Autodesk Fusion 360 part; units mm, degrees
note: some values were not read from the file. Chosen so that the rebuilt part matches the saved one: which bodies a step acts on; which face or edge a step refers to. Set by a fixed rule: which sketch regions a step uses.
(part 2 of 2)
sketch "Sketch34" plane through (0, 0, 200) normal (0, 0, 1) x (1, 0, 0)
  line L0 (263.504389, 9.486833) -> (116.666667, 450)
  line L1 (116.666667, 450) -> (-116.666667, 450)
  line L2 (-116.666667, 450) -> (-263.504389, 9.486833)
  arc A0 (-263.504394, 9.486818) -> (-235.04389, 0) centre (-249.27414, 4.743416) ccw
  line L3 (-235.04389, 0) -> (-135.04389, 300)
  line L4 (-135.04389, 300) -> (135.04389, 300)
  line L5 (135.04389, 300) -> (235.04389, 0)
  arc A1 (235.04389, 0) -> (263.504389, 9.486833) centre (249.27414, 4.743416) ccw
  line L6 (70, 350) -> (52.012308, 350)
  line L7 (52.012308, 350) -> (48.017663, 385.951807)
  line L8 (48.017663, 385.951807) -> (64.407497, 385.951807)
  line L9 (64.407497, 385.951807) -> (70, 350)
  line L10 (-47.987692, 350) -> (-43.993047, 385.951807)
  line L11 (-43.993047, 385.951807) -> (-27.603213, 385.951807)
  line L12 (-27.603213, 385.951807) -> (-30, 350)
  line L13 (-30, 350) -> (-47.987692, 350)
  line L14 (-43.548602, 389.951807) -> (-40.209914, 420)
  line L15 (-40.209914, 420) -> (-25.333333, 420)
  line L16 (-25.333333, 420) -> (-27.336546, 389.951807)
  line L17 (-27.336546, 389.951807) -> (-43.548602, 389.951807)
  line L18 (43.993047, 385.951807) -> (47.987692, 350)
  line L19 (47.987692, 350) -> (30, 350)
  line L20 (30, 350) -> (27.603213, 385.951807)
  line L21 (27.603213, 385.951807) -> (43.993047, 385.951807)
  line L22 (59.111111, 420) -> (63.785274, 389.951807)
  line L23 (63.785274, 389.951807) -> (47.573218, 389.951807)
  line L24 (47.573218, 389.951807) -> (44.23453, 420)
  line L25 (44.23453, 420) -> (59.111111, 420)
  line L26 (-64.407497, 385.951807) -> (-48.017663, 385.951807)
  line L27 (-48.017663, 385.951807) -> (-52.012308, 350)
  line L28 (-52.012308, 350) -> (-70, 350)
  line L29 (-70, 350) -> (-64.407497, 385.951807)
  line L30 (-63.785274, 389.951807) -> (-59.111111, 420)
  line L31 (-59.111111, 420) -> (-44.23453, 420)
  line L32 (-44.23453, 420) -> (-47.573218, 389.951807)
  line L33 (-47.573218, 389.951807) -> (-63.785274, 389.951807)
  line L34 (27.336546, 389.951807) -> (25.333333, 420)
  line L35 (25.333333, 420) -> (40.209914, 420)
  line L36 (40.209914, 420) -> (43.548602, 389.951807)
  line L37 (43.548602, 389.951807) -> (27.336546, 389.951807)
  line L38 (-235.04389, 0) -> (-263.504394, 9.486818)
  line L39 (-249.27414, 4.743416) -> (-254.017549, -9.486835)
  line L40 (-249.27414, 4.743416) -> (-150, 300)
  line L41 (-245.481053, 3.473564) -> (-146.208575, 298.725209)
  line L42 (-245.481053, 3.473564) -> (-250.222815, -10.751745)
  line L43 (-253.067226, 6.013269) -> (-153.791425, 301.274791)
  line L44 (-253.067226, 6.013269) -> (-257.812282, -8.221926)
  line L45 (-146.208575, 298.725209) -> (-144.574352, 303.585639)
  line L46 (-135.04389, 300) -> (-166.666667, 300)
  dimension "d166" = 4
  dimension "d167" = -4
  constraint parallel L41 L45
  constraint parallel L4 L46
extrude "Extrude30" cut sketch "Sketch34" along normal blind -5 and the other way blind 15 contours L38 L40 L43 L44 L46 | L38 L40 L41 L45 L46 picked at (-184.498063, 201.581139) picked at (-214.917844, 102.740639) bodies 11 12
extrude "Extrude31" cut 1 faces at (-181.826464, 201.1595, 195) along direction (0, 0, -1) blind 190 and the other way blind -180 on bodies 12 bodies 4 12
sketch "Sketch35" plane through (0, 300, 0) normal (0, -1, 0) x (1, 0, 0)
sketch "Sketch36" plane through (23.504389, -70.513167, 0) normal (-0.316228, 0.948683, 0) x (0, 0, 1)
  line L0 (190, 233.982213) -> (190, 241.984653)
  line L1 (190, 241.984653) -> (185, 241.984653)
  line L2 (185, 241.984653) -> (185, 233.982213)
  line L3 (185, 233.982213) -> (190, 233.982213)
  line L4 (15, 242.000004) -> (5, 242.000004)
  line L5 (5, 242.000004) -> (5, 234.000003)
  line L6 (5, 234.000003) -> (15, 234.000003)
  line L7 (15, 234.000003) -> (15, 242.000004)
  line L8 (185, 241.984653) -> (195.000003, 241.984653)
  line L9 (195.000003, 241.984653) -> (195.000003, 234.000003)
  line L10 (185, 234.000003) -> (185, 241.984653)
  constraint horizontal L4
  constraint vertical L5
  constraint horizontal L6
  constraint vertical L7
  constraint horizontal L8
  constraint vertical L9
  constraint vertical L10
extrude "Extrude32" cut sketch "Sketch36" 1 faces at (250.540594, 5.165568, 191.666667) along normal blind 340 and the other way blind 50 on bodies 12 bodies 9 10 12
sketch "Sketch37" plane through (-23.504315, -70.513069, 0) normal (0.316227, 0.948683, 0) x (0, 0, -1)
  line L0 (-190, 233.982238) -> (-190, 241.982252)
  line L1 (-190, 241.982252) -> (-195, 241.982252)
  line L2 (-195, 241.982252) -> (-195, 233.982238)
  line L3 (-195, 233.982238) -> (-190, 233.982238)
  line L4 (-5, 242.000004) -> (-15, 242.000004)
  line L5 (-15, 242.000004) -> (-15, 233.000003)
  line L6 (-15, 233.000003) -> (-5, 233.000003)
  line L7 (-5, 233.000003) -> (-5, 242.000004)
  line L8 (-185.000003, 242.000004) -> (-195.000003, 242.000004)
  line L9 (-195.000003, 242.000004) -> (-195.000003, 233.000003)
  line L10 (-195.000003, 233.000003) -> (-185.000003, 233.000003)
  line L11 (-185.000003, 233.000003) -> (-185.000003, 242.000004)
  constraint horizontal L4
  constraint vertical L5
  constraint horizontal L6
  constraint vertical L7
  constraint horizontal L8
  constraint vertical L9
  constraint horizontal L10
  constraint vertical L11
extrude "Extrude33" cut sketch "Sketch37" along normal blind 320 and the other way blind 60 bodies 4 11 12
